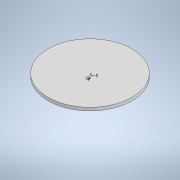
# Autodesk Inventor part: Soporte_mesa
Saved by Autodesk Inventor 2020 (Build 240168000, 168)
## iProperties
Created: 2023-03-22
Part Number: Soporte_mesa
Material: Generic
Document SubType Name: Modeling
Designer: semon
Density: 1 g/cm^3
Appearance: Default
Author: semon
Autodesk Inventor part; units mm, degrees
ref_plane "YZ Plane" through (0, 0, 0) normal (1, 0, 0) x (0, 1, 0)
ref_plane "XZ Plane" through (0, 0, 0) normal (0, 1, 0) x (-1, 0, 0)
ref_plane "XY Plane" through (0, 0, 0) normal (0, 0, 1) x (1, 0, 0)
sketch "Sketch1" plane through (0, 0, 0) normal (0, 1, 0) x (-1, 0, 0)
  circle A0 centre (0, 0) radius 4.5
  arc A1 (-1.5, 2) -> (1.5, 2) centre (0, 0) ccw
  line L0 (1.5, 2) -> (-1.5, 2)
  arc A2 (1.5, 2) -> (-1.5, 2) centre (0, 0) ccw construction
  dimension "d0" = 5
  dimension "d1" = 9
  dimension "d4" = 3
  constraints: 4 point on circle, 3 centre point, 2 coincident, 2 end point, 1 horizontal
  measures "d0" diameter of A1
  measures "d1" diameter of A0
  measures "d4" distance of L0.start L0.end
extrude "Extrusion1" add sketch "Sketch1" against normal blind 25
sketch "Sketch2" plane through (0, 0, 0) normal (0, -1, 0) x (-1, 0, 0)
  circle A0 centre (0, 0) radius 40
  dimension "d5" = 80
  constraints: 1 centre point, 1 coincident
  measures "d5" diameter of A0
extrude "Extrusion2" add sketch "Sketch2" against normal blind 3
extrude "Extrusion3" add sketch "Sketch1" against normal blind 5 contours L0 A1
body "Solid1"
